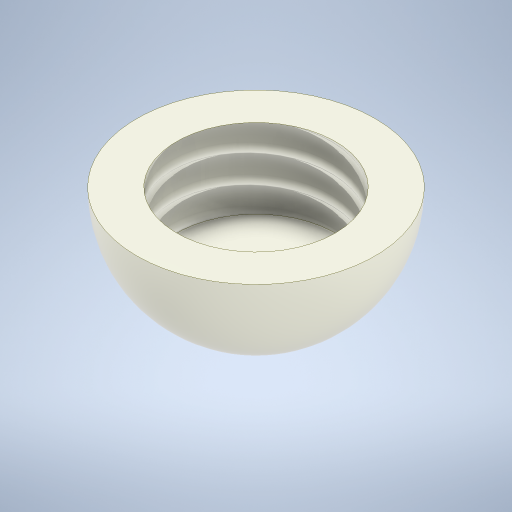
# Autodesk Inventor part: transversal_stab_tip
Saved by Autodesk Inventor 2024 (Build 280153000, 153)
## iProperties
Created: 2025-12-17
Part Number: transversal_stab_tip
Material: Polytetrafluoroethylene
Document SubType Name: Modeling
Designer: schar
Density: 2.02 g/cm^3
Appearance: Smooth - Ivory
Author: schar
Autodesk Inventor part; units mm, degrees
ref_plane "YZ Plane" through (0, 0, 0) normal (1, 0, 0) x (0, 1, 0)
ref_plane "XZ Plane" through (0, 0, 0) normal (0, 1, 0) x (-1, 0, 0)
ref_plane "XY Plane" through (0, 0, 0) normal (0, 0, 1) x (1, 0, 0)
sketch "Sketch1" plane through (0, 0, 0) normal (1, 0, 0) x (0, 1, 0)
  line L0 (0, 0) -> (0, -3)
  line L1 (0, 0) -> (-3, 0)
  line L2 (0, 0) -> (0, 5)
  circle A0 centre (0, 0) radius 3
  point P0 (0, 3)
  dimension "d0" = 3
  dimension "d1" = 3
  dimension "d2" = 5
  constraints: 6 end point, 2 vertical, 1 coincident, 1 horizontal, 3 other
  measures "d0" distance of L0.start L0.end
  measures "d1" distance of L0.start L1.end
  measures "d2" distance of L0.start L2.end
revolve "Revolution1" add sketch "Sketch1" angle 360 about axis through (0, 0, 0) along (0, -1, 0) contours L1 A0 L2
sketch "Sketch2" plane through (0, 0, 0) normal (0, 1, 0) x (1, 0, 0)
  circle A0 centre (0, 0) radius 2
  dimension "d4" = 4
  constraints: 1 centre point, 1 coincident
  measures "d4" diameter of A0
extrude "Extrusion1" cut sketch "Sketch2" against normal blind 2
thread "Thread1" size "M4x0.7" class "6H" standard "ANSI Metric M Profile" length 70
body "Solid1"
